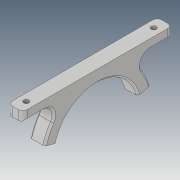
# Autodesk Inventor part: bottomCameraMount
Saved by Autodesk Inventor 2018 (Build 220112000, 112)
## iProperties
Created: 2020-01-25
Part Number: bottomCameraMount
Material: Generic
Document SubType Name: Modeling
Designer: anirudh
Density: 1 g/cm^3
Appearance: Default
Author: anirudh
Autodesk Inventor part; units mm, degrees
ref_plane "YZ Plane" through (0, 0, 0) normal (1, 0, 0) x (0, 1, 0)
ref_plane "XZ Plane" through (0, 0, 0) normal (0, 1, 0) x (-1, 0, 0)
ref_plane "XY Plane" through (0, 0, 0) normal (0, 0, 1) x (1, 0, 0)
sketch "Sketch1" plane through (0, 0, 0) normal (1, 0, 0) x (0, 1, 0)
  arc A0 (7.3958, -27.6013) -> (7.3958, 27.6013) centre (0, 0) ccw
  line L0 (7.3958, 27.6013) -> (9.6178, 35.894)
  line L1 (0, 0) -> (46.4224, 0) construction
  line L2 (7.3958, -27.6013) -> (9.6178, -35.894)
  line L3 (0, 0) -> (51.2466, 0) construction
  line L4 (30.8102, 20.7753) -> (30.8102, 50.8)
  line L5 (30.8102, 50.8) -> (37.1602, 50.8)
  line L6 (37.1602, 50.8) -> (37.1602, 0)
  line L7 (37.1602, 0) -> (37.1602, -50.8)
  line L8 (37.1602, -50.8) -> (30.8102, -50.8)
  line L9 (30.8102, -50.8) -> (30.8102, -20.7753)
  arc A1 (9.6178, -35.894) -> (30.8102, -20.7753) centre (0, 0) ccw
  arc A2 (30.8102, 20.7753) -> (9.6178, 35.894) centre (0, 0) ccw
  constraints: 20 end point, 6 point on circle, 4 perpendicular, 3 centre point, 3 point on line, 2 coincident, 2 horizontal
extrude "Extrusion1" add sketch "Sketch1" along normal blind 10.16
sketch "Sketch2" plane through (0, 30.8102, 20.7753) normal (0, -1, 0) x (1, 0, 0)
  line L0 (0, 15.1187) -> (10.16, 15.1187)
  line L1 (10.16, -48.3766) -> (10.16, -56.6693) projected
  line L2 (10.16, 15.1187) -> (10.16, 6.8261) projected
  circle A0 centre (5.08, 22.5717) radius 1.75
  circle A1 centre (5.08, -64.1223) radius 1.75
  point P0 (0, -20.7753)
  point P1 (10.16, 30.0247)
  point P2 (0, 30.0247)
  point P3 (0, -71.5753)
  dimension "d10" = 3.5
  dimension "d11" = 3.5
  constraints: 2 centre point, 2 end point
  measures "d10" diameter of A0
  measures "d11" diameter of A1
extrude "Extrusion2" cut sketch "Sketch2" against normal blind 10.16
sketch "Sketch3" plane through (0, 7.3958, 27.6013) normal (0, -0.9659, 0.2588) x (1, 0, 0)
  circle A0 centre (5.08, 4.2926) radius 2.2
  point P0 (0, -28.575)
  point P1 (0, 8.5852)
  point P2 (10.16, 0)
  dimension "d16" = 4.4
  constraints: 1 centre point
  measures "d16" diameter of A0
extrude "Extrusion3" cut sketch "Sketch3" against normal blind 4.8
sketch "Sketch4" plane through (0, 9.6178, -35.894) normal (0, -0.9659, -0.2588) x (1, 0, 0)
  circle A0 centre (5.08, 4.2926) radius 2.2
  point P0 (0, 37.1602)
  point P1 (0, 0)
  point P2 (10.16, 8.5852)
  constraints: 1 centre point
extrude "Extrusion4" cut sketch "Sketch4" against normal blind 4.8
fillet "Fillet1" radius 6.35 2 edges at (5.08, 30.8102, -20.7753) (5.08, 30.8102, 20.7753)
chamfer "Chamfer2" distance 1.27 angle 45 10 edges at (10.16, 15.4709, 33.7866) (10.16, 30.8102, 43.3919) (0, 15.4709, 33.7866) (0, 30.8102, 43.3919) (0, 28.575, 0) (10.16, 28.575, 0) (10.16, 15.4709, -33.7866) (10.16, 30.8102, -43.3919) (0, 15.4709, -33.7866) (0, 30.8102, -43.3919)
fillet "Fillet2" radius 3.175 4 edges at (0, 34.6202, 50.8) (10.16, 34.6202, 50.8) (0, 34.6202, -50.8) (10.16, 34.6202, -50.8)
body "Solid1"
